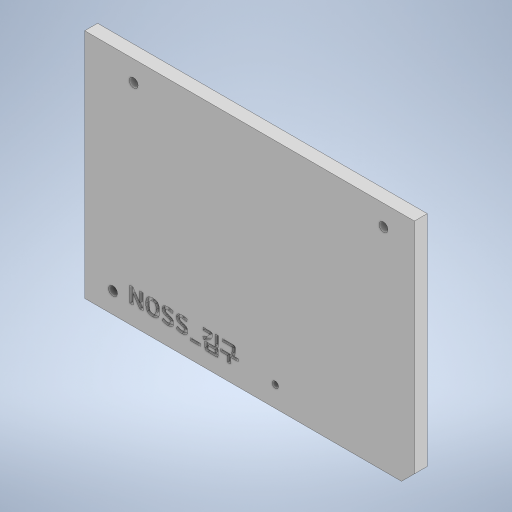
# Autodesk Inventor part: 아크릴 커버
Saved by Autodesk Inventor 2023 (Build 270158000, 158)
## iProperties
Created: 2022-11-10
Part Number: 아크릴 커버
Material: 일반
Document SubType Name: Modeling
Designer: user
Density: 1 g/cm^3
Appearance: 기본값
Author: user
Autodesk Inventor part; units mm, degrees
ref_plane "YZ Plane" through (0, 0, 0) normal (1, 0, 0) x (0, 1, 0)
ref_plane "XZ Plane" through (0, 0, 0) normal (0, 1, 0) x (-1, 0, 0)
ref_plane "XY Plane" through (0, 0, 0) normal (0, 0, 1) x (1, 0, 0)
sketch "스케치1" plane through (0, 0, 0) normal (0, 0, 1) x (1, 0, 0)
  line L0 (-64, 45) -> (64, 45)
  line L1 (64, 45) -> (64, -40)
  line L2 (59, -45) -> (-64, -45)
  line L3 (-64, -45) -> (-64, 45)
  line L4 (-64, 45) -> (64, -45) construction
  line L5 (64, 45) -> (-64, -45) construction
  line L6 (59, -45) -> (64, -40)
  circle A0 centre (-53, -37) radius 1.75
  circle A1 centre (10, -37) radius 1.25
  circle A2 centre (-45, 37) radius 1.75
  circle A3 centre (52, 37) radius 1.75
  point P0 (0, 0)
  dimension "d0" = 128
  dimension "d1" = 90
  dimension "d2" = 5
  dimension "d3" = 5
  dimension "d4" = 3.5
  dimension "d5" = 2.5
  dimension "d6" = 3.5
  dimension "d7" = 3.5
  dimension "d8" = 19
  dimension "d9" = 97
  dimension "d10" = 8
  dimension "d11" = 63
  dimension "d12" = 11
  dimension "d13" = 8
  constraints: 14 end point, 4 centre point, 2 horizontal alignment, 2 midpoint, 2 parallel, 2 point on line, 1 horizontal, 1 perpendicular
  measures "d0" distance of L0.start L0.end
  measures "d1" distance of L0.end L4.end
  measures "d2" distance of L2.start L4.end
  measures "d3" distance of L1.end L4.end
  measures "d4" diameter of A0
  measures "d5" diameter of A1
  measures "d6" diameter of A2
  measures "d7" diameter of A3
  measures "d8" distance from line of L3 A2.centre
  measures "d9" distance of A3.centre A2.centre
  measures "d10" distance from line of L0 A2.centre
  measures "d11" distance of A1.centre A0.centre
  measures "d12" distance from line of L3 A0.centre
  measures "d13" distance from line of L2 A0.centre
extrude "돌출1" add sketch "스케치1" along normal blind 5
sketch "스케치2" plane through (0, 0, 5) normal (0, 0, 1) x (1, 0, 0)
  line L0 (-47.0595, -31.626) -> (-4.2188, -31.626) construction
  line L1 (-4.2188, -31.626) -> (-4.2188, -39.0601) construction
  line L2 (-4.2188, -39.0601) -> (-47.0595, -39.0601) construction
  line L3 (-47.0595, -39.0601) -> (-47.0595, -31.626) construction
  line L4 (-46.4702, -31.8197) -> (-46.462, -37.8197)
  line L5 (-46.462, -37.8197) -> (-45.201, -37.8197)
  line L6 (-45.201, -37.8197) -> (-45.201, -33.9213)
  line L7 (-45.201, -33.9213) -> (-42.6296, -37.8197)
  line L8 (-42.6296, -37.8197) -> (-41.3644, -37.8197)
  line L9 (-41.3644, -37.8197) -> (-41.3644, -31.8197)
  line L10 (-41.3644, -31.8197) -> (-42.6296, -31.8197)
  line L11 (-42.6296, -31.8197) -> (-42.6296, -35.7757)
  line L12 (-42.6296, -35.7757) -> (-45.2381, -31.8197)
  line L13 (-45.2381, -31.8197) -> (-46.4702, -31.8197)
  spline S0 degree 2 poles (-34.9318, -34.8733) (-34.9318, -34.0985) (-35.1749, -32.9076) (-35.4716, -32.5038) knots 0 0 0 1 2 2 2
  spline S1 degree 2 poles (-35.4716, -32.5038) (-35.7765, -32.104) (-36.8026, -31.6919) (-37.598, -31.6919) knots 0 0 0 1 2 2 2
  spline S2 degree 2 poles (-37.598, -31.6919) (-38.3892, -31.6919) (-39.4194, -32.1164) (-39.7243, -32.512) knots 0 0 0 1 2 2 2
  spline S3 degree 2 poles (-39.7243, -32.512) (-40.0293, -32.8994) (-40.2642, -34.0491) (-40.2642, -34.7661) knots 0 0 0 1 2 2 2
  spline S4 degree 2 poles (-40.2642, -34.7661) (-40.2642, -35.5656) (-40.0128, -36.7565) (-39.7079, -37.1521) knots 0 0 0 1 2 2 2
  spline S5 degree 2 poles (-39.7079, -37.1521) (-39.3947, -37.5477) (-38.3727, -37.9392) (-37.6062, -37.9392) knots 0 0 0 1 2 2 2
  spline S6 degree 2 poles (-37.6062, -37.9392) (-36.8644, -37.9392) (-35.8342, -37.5683) (-35.521, -37.1768) knots 0 0 0 1 2 2 2
  spline S7 degree 2 poles (-35.521, -37.1768) (-35.2079, -36.7977) (-34.9318, -35.6521) (-34.9318, -34.8733) knots 0 0 0 1 2 2 2
  spline S8 degree 2 poles (-37.598, -36.9255) (-38.3068, -36.9255) (-38.9496, -35.9818) (-38.9496, -34.7661) knots 0 0 0 1 2 2 2
  spline S9 degree 2 poles (-38.9496, -34.7661) (-38.9496, -34.181) (-38.7807, -33.398) (-38.6117, -33.1507) knots 0 0 0 1 2 2 2
  spline S10 degree 2 poles (-38.6117, -33.1507) (-38.4427, -32.9158) (-37.9359, -32.7057) (-37.598, -32.7057) knots 0 0 0 1 2 2 2
  spline S11 degree 2 poles (-37.598, -32.7057) (-37.2436, -32.7057) (-36.7367, -32.9241) (-36.5677, -33.1796) knots 0 0 0 1 2 2 2
  spline S12 degree 2 poles (-36.5677, -33.1796) (-36.407, -33.431) (-36.2463, -34.2593) (-36.2463, -34.8733) knots 0 0 0 1 2 2 2
  spline S13 degree 2 poles (-36.2463, -34.8733) (-36.2463, -36.0395) (-36.9386, -36.9255) (-37.598, -36.9255) knots 0 0 0 1 2 2 2
  spline S14 degree 2 poles (-31.7834, -36.9255) (-32.0265, -36.9255) (-32.4427, -36.8224) (-32.6447, -36.7483) knots 0 0 0 1 2 2 2
  spline S15 degree 2 poles (-32.6447, -36.7483) (-32.8466, -36.67) (-33.2752, -36.4763) (-33.5142, -36.3609) knots 0 0 0 1 2 2 2
  line L14 (-33.5142, -36.3609) -> (-33.918, -37.3623)
  spline S16 degree 2 poles (-33.918, -37.3623) (-33.3699, -37.6425) (-32.3068, -37.9474) (-31.7834, -37.9474) knots 0 0 0 1 2 2 2
  spline S17 degree 2 poles (-31.7834, -37.9474) (-30.5677, -37.9474) (-29.4304, -36.9502) (-29.4304, -36.0807) knots 0 0 0 1 2 2 2
  spline S18 degree 2 poles (-29.4304, -36.0807) (-29.4304, -35.7098) (-29.6488, -35.1865) (-29.8425, -35.001) knots 0 0 0 1 2 2 2
  spline S19 degree 2 poles (-29.8425, -35.001) (-30.0279, -34.8156) (-30.5348, -34.5601) (-30.8191, -34.4612) knots 0 0 0 1 2 2 2
  spline S20 degree 2 poles (-30.8191, -34.4612) (-30.9881, -34.4117) (-31.2601, -34.3087) (-31.396, -34.2593) knots 0 0 0 1 2 2 2
  spline S21 degree 2 poles (-31.396, -34.2593) (-31.532, -34.2057) (-31.8329, -34.0985) (-32.0265, -34.0202) knots 0 0 0 1 2 2 2
  spline S22 degree 2 poles (-32.0265, -34.0202) (-32.3068, -33.9213) (-32.6035, -33.6576) (-32.6035, -33.431) knots 0 0 0 1 2 2 2
  spline S23 degree 2 poles (-32.6035, -33.431) (-32.6035, -33.126) (-32.146, -32.7057) (-31.6392, -32.7057) knots 0 0 0 1 2 2 2
  spline S24 degree 2 poles (-31.6392, -32.7057) (-31.293, -32.7057) (-30.5842, -32.9323) (-30.0032, -33.1507) knots 0 0 0 1 2 2 2
  line L15 (-30.0032, -33.1507) -> (-29.7147, -32.1658)
  spline S25 degree 2 poles (-29.7147, -32.1658) (-30.2216, -31.9392) (-31.2188, -31.6919) (-31.6392, -31.6919) knots 0 0 0 1 2 2 2
  spline S26 degree 2 poles (-31.6392, -31.6919) (-32.1131, -31.6919) (-32.9414, -31.8856) (-33.2422, -32.0958) knots 0 0 0 1 2 2 2
  spline S27 degree 2 poles (-33.2422, -32.0958) (-33.5471, -32.3101) (-33.9015, -32.9571) (-33.9015, -33.4227) knots 0 0 0 1 2 2 2
  spline S28 degree 2 poles (-33.9015, -33.4227) (-33.9015, -34.1068) (-33.2504, -34.7908) (-32.5952, -35.0175) knots 0 0 0 1 2 2 2
  spline S29 degree 2 poles (-32.5952, -35.0175) (-32.3727, -35.104) (-32.0554, -35.2112) (-31.9194, -35.2606) knots 0 0 0 1 2 2 2
  spline S30 degree 2 poles (-31.9194, -35.2606) (-31.7834, -35.3142) (-31.5197, -35.4131) (-31.3425, -35.4749) knots 0 0 0 1 2 2 2
  spline S31 degree 2 poles (-31.3425, -35.4749) (-31.2518, -35.5161) (-31.0499, -35.6068) (-30.9633, -35.6768) knots 0 0 0 1 2 2 2
  spline S32 degree 2 poles (-30.9633, -35.6768) (-30.8727, -35.7428) (-30.7614, -35.9447) (-30.7532, -36.0889) knots 0 0 0 1 2 2 2
  spline S33 degree 2 poles (-30.7532, -36.0889) (-30.7532, -36.4186) (-31.2106, -36.9419) (-31.7834, -36.9255) knots 0 0 0 1 2 2 2
  spline S34 degree 2 poles (-26.282, -36.9255) (-26.5252, -36.9255) (-26.9414, -36.8224) (-27.1433, -36.7483) knots 0 0 0 1 2 2 2
  spline S35 degree 2 poles (-27.1433, -36.7483) (-27.3452, -36.67) (-27.7738, -36.4763) (-28.0128, -36.3609) knots 0 0 0 1 2 2 2
  line L16 (-28.0128, -36.3609) -> (-28.4166, -37.3623)
  spline S36 degree 2 poles (-28.4166, -37.3623) (-27.8686, -37.6425) (-26.8054, -37.9474) (-26.282, -37.9474) knots 0 0 0 1 2 2 2
  spline S37 degree 2 poles (-26.282, -37.9474) (-25.0664, -37.9474) (-23.929, -36.9502) (-23.929, -36.0807) knots 0 0 0 1 2 2 2
  spline S38 degree 2 poles (-23.929, -36.0807) (-23.929, -35.7098) (-24.1474, -35.1865) (-24.3411, -35.001) knots 0 0 0 1 2 2 2
  spline S39 degree 2 poles (-24.3411, -35.001) (-24.5265, -34.8156) (-25.0334, -34.5601) (-25.3177, -34.4612) knots 0 0 0 1 2 2 2
  spline S40 degree 2 poles (-25.3177, -34.4612) (-25.4867, -34.4117) (-25.7587, -34.3087) (-25.8947, -34.2593) knots 0 0 0 1 2 2 2
  spline S41 degree 2 poles (-25.8947, -34.2593) (-26.0307, -34.2057) (-26.3315, -34.0985) (-26.5252, -34.0202) knots 0 0 0 1 2 2 2
  spline S42 degree 2 poles (-26.5252, -34.0202) (-26.8054, -33.9213) (-27.1021, -33.6576) (-27.1021, -33.431) knots 0 0 0 1 2 2 2
  spline S43 degree 2 poles (-27.1021, -33.431) (-27.1021, -33.126) (-26.6447, -32.7057) (-26.1378, -32.7057) knots 0 0 0 1 2 2 2
  spline S44 degree 2 poles (-26.1378, -32.7057) (-25.7916, -32.7057) (-25.0829, -32.9323) (-24.5018, -33.1507) knots 0 0 0 1 2 2 2
  line L17 (-24.5018, -33.1507) -> (-24.2133, -32.1658)
  spline S45 degree 2 poles (-24.2133, -32.1658) (-24.7202, -31.9392) (-25.7175, -31.6919) (-26.1378, -31.6919) knots 0 0 0 1 2 2 2
  spline S46 degree 2 poles (-26.1378, -31.6919) (-26.6117, -31.6919) (-27.44, -31.8856) (-27.7408, -32.0958) knots 0 0 0 1 2 2 2
  spline S47 degree 2 poles (-27.7408, -32.0958) (-28.0458, -32.3101) (-28.4002, -32.9571) (-28.4002, -33.4227) knots 0 0 0 1 2 2 2
  spline S48 degree 2 poles (-28.4002, -33.4227) (-28.4002, -34.1068) (-27.7491, -34.7908) (-27.0938, -35.0175) knots 0 0 0 1 2 2 2
  spline S49 degree 2 poles (-27.0938, -35.0175) (-26.8713, -35.104) (-26.554, -35.2112) (-26.418, -35.2606) knots 0 0 0 1 2 2 2
  spline S50 degree 2 poles (-26.418, -35.2606) (-26.282, -35.3142) (-26.0183, -35.4131) (-25.8411, -35.4749) knots 0 0 0 1 2 2 2
  spline S51 degree 2 poles (-25.8411, -35.4749) (-25.7504, -35.5161) (-25.5485, -35.6068) (-25.462, -35.6768) knots 0 0 0 1 2 2 2
  spline S52 degree 2 poles (-25.462, -35.6768) (-25.3713, -35.7428) (-25.2601, -35.9447) (-25.2518, -36.0889) knots 0 0 0 1 2 2 2
  spline S53 degree 2 poles (-25.2518, -36.0889) (-25.2518, -36.4186) (-25.7092, -36.9419) (-26.282, -36.9255) knots 0 0 0 1 2 2 2
  line L18 (-19.0746, -37.6672) -> (-22.9153, -37.6672)
  line L19 (-22.9153, -37.6672) -> (-22.9153, -38.6315)
  line L20 (-22.9153, -38.6315) -> (-19.0746, -38.6315)
  line L21 (-19.0746, -38.6315) -> (-19.0746, -37.6672)
  spline S54 degree 2 poles (-12.1351, -36.7647) (-12.1103, -36.4351) (-12.3205, -36.0724) (-12.5513, -36.0065) knots 0 0 0 1 2 2 2
  spline S55 degree 2 poles (-12.5513, -36.0065) (-12.3576, -35.8623) (-12.0938, -35.3719) (-12.0938, -35.034) knots 0 0 0 1 2 2 2
  line L22 (-12.0938, -35.034) -> (-12.0938, -31.626)
  line L23 (-12.0938, -31.626) -> (-13.3095, -31.626)
  line L24 (-13.3095, -31.626) -> (-13.3095, -35.1205)
  spline S56 degree 2 poles (-13.3095, -35.1205) (-13.3095, -35.3719) (-13.4455, -35.8293) (-13.5897, -35.9694) knots 0 0 0 1 2 2 2
  line L25 (-13.5897, -35.9694) -> (-17.3026, -35.9694)
  line L26 (-17.3026, -35.9694) -> (-17.3026, -38.1741)
  spline S57 degree 2 poles (-17.3026, -38.1741) (-17.3026, -38.7057) (-16.771, -39.0601) (-16.2394, -39.0601) knots 0 0 0 1 2 2 2
  line L27 (-16.2394, -39.0601) -> (-12.7614, -39.0601)
  spline S58 degree 2 poles (-12.7614, -39.0601) (-12.543, -39.0601) (-12.2875, -38.8994) (-12.271, -38.7139) knots 0 0 0 1 2 2 2
  line L28 (-12.271, -38.7139) -> (-12.1351, -36.7647)
  line L29 (-18.0361, -32.6892) -> (-15.7573, -32.6892)
  spline S59 degree 2 poles (-15.7573, -32.6892) (-15.6749, -32.6892) (-15.5471, -32.7881) (-15.5966, -32.9323) knots 0 0 0 1 2 2 2
  spline S60 degree 2 poles (-15.5966, -32.9323) (-15.7161, -33.2373) (-16.2147, -33.7771) (-16.5609, -34.012) knots 0 0 0 1 2 2 2
  spline S61 degree 2 poles (-16.5609, -34.012) (-16.907, -34.251) (-17.723, -34.6466) (-18.1474, -34.8073) knots 0 0 0 1 2 2 2
  line L30 (-18.1474, -34.8073) -> (-17.69, -35.7263)
  spline S62 degree 2 poles (-17.69, -35.7263) (-17.0059, -35.4667) (-15.8232, -34.8485) (-15.3699, -34.4694) knots 0 0 0 1 2 2 2
  spline S63 degree 2 poles (-15.3699, -34.4694) (-14.9208, -34.0903) (-14.3809, -33.159) (-14.3397, -32.5944) knots 0 0 0 1 2 2 2
  spline S64 degree 2 poles (-14.3397, -32.5944) (-14.315, -32.1906) (-14.6282, -31.7414) (-15.0073, -31.7414) knots 0 0 0 1 2 2 2
  line L31 (-15.0073, -31.7414) -> (-18.0361, -31.7414)
  line L32 (-18.0361, -31.7414) -> (-18.0361, -32.6892)
  spline S65 degree 2 poles (-15.8933, -38.1082) (-16.0169, -38.1082) (-16.087, -38.0134) (-16.087, -37.8856) knots 0 0 0 1 2 2 2
  line L33 (-16.087, -37.8856) -> (-16.087, -36.9172)
  line L34 (-16.087, -36.9172) -> (-13.3878, -36.9172)
  line L35 (-13.3878, -36.9172) -> (-13.3878, -38.1082)
  line L36 (-13.3878, -38.1082) -> (-15.8933, -38.1082)
  line L37 (-7.359, -38.7634) -> (-7.359, -36.4516)
  line L38 (-7.359, -36.4516) -> (-4.429, -36.4516)
  line L39 (-4.429, -36.4516) -> (-4.429, -35.5079)
  line L40 (-4.429, -35.5079) -> (-11.1831, -35.5079)
  line L41 (-11.1831, -35.5079) -> (-11.1831, -36.4516)
  line L42 (-11.1831, -36.4516) -> (-8.5993, -36.4516)
  line L43 (-8.5993, -36.4516) -> (-8.5993, -38.7634)
  line L44 (-8.5993, -38.7634) -> (-7.359, -38.7634)
  spline S66 degree 2 poles (-5.8136, -35.2194) (-5.6529, -34.5354) (-5.451, -33.262) (-5.4427, -32.6191) knots 0 0 0 1 2 2 2
  spline S67 degree 2 poles (-5.4427, -32.6191) (-5.4427, -32.2483) (-5.8219, -31.795) (-6.304, -31.795) knots 0 0 0 1 2 2 2
  line L45 (-6.304, -31.795) -> (-10.4826, -31.795)
  line L46 (-10.4826, -31.795) -> (-10.4826, -32.7304)
  line L47 (-10.4826, -32.7304) -> (-6.9386, -32.7304)
  spline S68 degree 2 poles (-6.9386, -32.7304) (-6.8109, -32.7304) (-6.6666, -32.8829) (-6.6666, -33.0354) knots 0 0 0 1 2 2 2
  spline S69 degree 2 poles (-6.6666, -33.0354) (-6.6666, -33.4886) (-6.8356, -34.6219) (-6.9386, -35.0834) knots 0 0 0 1 2 2 2
  line L48 (-6.9386, -35.0834) -> (-5.8136, -35.2194)
  point P0 (0, 0)
  constraints: 2 other
extrude "돌출2" cut sketch "스케치2" against normal blind 1
equation "\"d3\" = d2"
